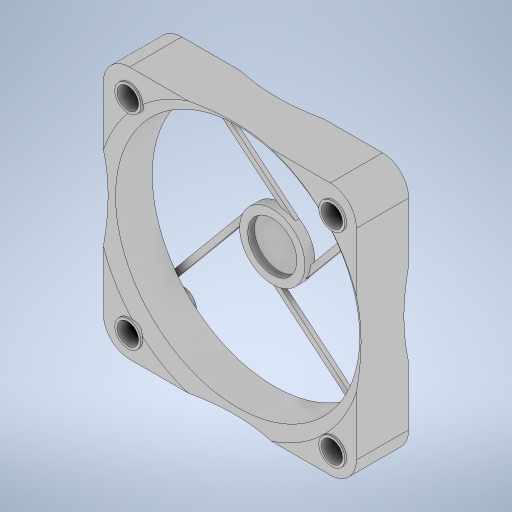
# Autodesk Inventor part: Suporte da Ventoinha
Saved by Autodesk Inventor 2023.2 (Build 272271000, 271)
## iProperties
Created: 2022-12-15
Part Number: Suporte da Ventoinha
Material: Generic
Document SubType Name: Sheet Metal
Designer: coqui
Density: 1 g/cm^3
Sheet Metal Rule: Default_mm
Appearance: Default
Author: coqui
Autodesk Inventor part; units mm, degrees
ref_plane "YZ Plane" through (0, 0, 0) normal (1, 0, 0) x (0, 1, 0)
ref_plane "XZ Plane" through (0, 0, 0) normal (0, 1, 0) x (-1, 0, 0)
sketch "Sketch3" plane through (0, 0, 0) normal (0, 0, 1) x (1, 0, 0)
  line L0 (-61.5, 77.5) -> (61.5, 77.5)
  line L1 (77.5, 61.5) -> (77.5, -61.5)
  line L2 (61.5, -77.5) -> (-61.5, -77.5)
  line L3 (-77.5, -61.5) -> (-77.5, 61.5)
  line L4 (-77.5, 77.5) -> (77.5, -77.5) construction
  line L5 (77.5, 77.5) -> (-77.5, -77.5) construction
  arc A0 (-61.5, 77.5) -> (-77.5, 61.5) centre (-61.5, 61.5) ccw
  arc A1 (-77.5, -61.5) -> (-61.5, -77.5) centre (-61.5, -61.5) ccw
  arc A2 (61.5, -77.5) -> (77.5, -61.5) centre (61.5, -61.5) ccw
  arc A3 (77.5, 61.5) -> (61.5, 77.5) centre (61.5, 61.5) ccw
  circle A4 centre (-61.5, 61.5) radius 6.5
  circle A5 centre (63.5, 61.5) radius 6.5
  circle A6 centre (-61.5, -63.5) radius 6.5
  circle A7 centre (63.5, -63.5) radius 6.5
  point P0 (0, 0)
  dimension "d29" = 155
  dimension "d30" = 155
  dimension "d31" = 16
  dimension "d33" = 13
  dimension "d36" = 125
  dimension "d39" = 125
  constraints: 12 end point, 8 centre point, 8 point on circle, 8 point on line, 8 tangent, 3 equal radius, 2 horizontal, 2 midpoint, 2 parallel, 1 coincident, 1 perpendicular, 1 vertical, 6 other
  measures "d29" distance of L5.start L4.end
  measures "d30" distance of L4.start L5.start
  measures "d31" radius of A0
  measures "d33" diameter of A4
  measures "d36" distance of A4.centre A5.centre
  measures "d39" distance of A4.centre A6.centre
extrude "Extrusion2" add sketch "Sketch3" along normal mid plane 32
sketch "Sketch4" plane through (0, 0, 0) normal (0, 1, 0) x (-1, 0, 0)
  line L0 (0, -17) -> (0, 17)
  line L1 (0, 17) -> (-83, 17)
  line L2 (-83, 17) -> (-74.7881, 11.25)
  line L3 (-74.7881, 11.25) -> (-74.7881, -11.25)
  line L4 (-74.7881, -11.25) -> (-83, -17)
  line L5 (-83, -17) -> (0, -17)
  line L6 (-61.5, -16) -> (61.5, -16) projected
  line L7 (0, 45.4211) -> (0, -37.6603) construction
  point P0 (0, 0)
  point P1 (0, -16)
  point P2 (0, 0)
  dimension "d46" = 22.5
  dimension "d50" = 34
  dimension "d55" = 34
  dimension "d56" = 125
  dimension "d57" = 125
  dimension "d58" = 17
  dimension "d59" = 83
  dimension "d60" = 83
  dimension "d61" = 74.7882
  constraints: 14 end point, 2 midpoint, 2 parallel, 2 vertical, 1 perpendicular
  measures "d46" distance of L2.end L3.end
  measures "d50" distance of L4.end L1.end
  measures "d55" distance of L0.end L0.start
  measures "d56" angle of L2 L3
  measures "d57" angle of L3 L4
  measures "d58" vertical distance of point (0, 0) L4.end
  measures "d59" horizontal distance of point (0, 0) L1.end
  measures "d60" horizontal distance of point (0, 0) L4.end
  measures "d61" horizontal distance of point (0, 0) L2.end
revolve "Revolution2" cut sketch "Sketch4" angle 360 about axis through (0, 0, 45.4211) along (0, 0, -1)
sketch "Sketch6" plane through (0, 0, 0) normal (0, 0, 1) x (1, 0, 0)
  circle A0 centre (-61.5, -63.5) radius 6.5 projected
  circle A1 centre (-61.5, -63.5) radius 8
  circle A2 centre (-61.5, -63.5) radius 6.5
  point P0 (0, 0)
  dimension "d62" = 16
  dimension "d63" = 13
  constraints: 2 centre point, 2 coincident
  measures "d62" diameter of A1
  measures "d63" diameter of A2
extrude "Extrusion3" add sketch "Sketch6" along normal mid plane 34
pattern_linear "Rectangular Pattern1" count 2 spacing 125 along (0, 1, 0) count 2 spacing 125 along (1, 0, 0) of "Extrusion3"
sketch "Sketch10" plane through (0, 0, -16) normal (0, 0, -1) x (-1, 0, 0)
  circle A0 centre (0, 0) radius 20
  dimension "d79" = 40
  constraints: 1 centre point, 1 coincident
  measures "d79" diameter of A0
extrude "Extrusion6" add sketch "Sketch10" against normal blind 6
sketch "Sketch11" plane through (0, 0, -10) normal (0, 0, 1) x (1, 0, 0)
  circle A0 centre (0, 0) radius 15
  dimension "d82" = 30
  constraints: 1 centre point, 1 coincident
  measures "d82" diameter of A0
extrude "Extrusion7" cut sketch "Sketch11" against normal blind 4
sketch "Sketch12" plane through (0, 0, -16) normal (0, 0, -1) x (-1, 0, 0)
  circle A0 centre (0, 0) radius 20 projected
  line L0 (17.0488, 10.4566) -> (64.234, -46.2624)
  constraints: 2 end point, 2 other
ref_plane "Work Plane1" through (-64.234, -46.2624, -16) normal (-0.6395399, -0.7687579, 0) x (0.7687579, -0.6395399, 0)
sketch "Sketch16" plane through (-64.234, -46.2624, -16) normal (-0.6395399, -0.7687579, 0) x (0.7687579, -0.6395399, 0)
  line L0 (0, 0) -> (3.5, 0)
  line L1 (3.5, 0) -> (3.5, 2.5)
  line L2 (3.5, 2.5) -> (0, 2.5)
  line L3 (0, 2.5) -> (0, 0)
  point P0 (19.7938, 16)
  dimension "d88" = 3.5
  dimension "d89" = 2.5
  constraints: 8 end point, 2 horizontal, 2 parallel, 1 perpendicular, 1 vertical
  measures "d88" distance of L2.end L1.end
  measures "d89" distance of L0.end L1.end
sweep "Sweep1" add profiles "Sketch16" path "Sketch12" path curves L0
sketch "Sketch18" plane through (-61.5434, -48.5008, -16) normal (-0.6395399, -0.7687579, 0) x (0.7687579, -0.6395399, 0)
  spline S0 degree 2 poles (-3.5, 1.6892) (-1.7411, 1.9971) (0, 2.2506) knots 0 0 0 1 1 1 weights 1 1.000247 1 projected
  line L0 (-3.5, 1.6892) -> (-3.5, 0) projected
  line L1 (-3.5, 0) -> (0, 0) projected
  line L2 (0, 0) -> (0, 2.2506) projected
  point P0 (16.2938, 16)
  constraints: 1 other
extrude "Extrusion8" add sketch "Sketch18" along normal blind 6.25
pattern_circular "Circular Pattern1" count 4 over 360 about axis through (0, 0, -16) along (0, 0, 1) of "Sweep1", "Extrusion8"
equation "\"BendRadius\" = Thickness"
equation "\"BendReliefWidth\" = Thickness"
equation "\"BendReliefDepth\" = 0.5 * Thickness"
equation "\"CornerReliefSize\" = 4 * Thickness"
equation "\"MinimumRemnant\" = 2 * Thickness"
equation "\"TransitionRadius\" = BendRadius"
equation "\"JacobiRadiusSize\" = BendRadius"
equation "\"GapSize\" = Thickness"
equation "\"Thickness\" = 0.5"
body "Solid2"
